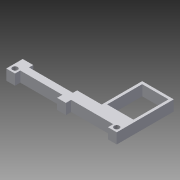
# Autodesk Inventor part: yCarMid_d
Saved by Autodesk Inventor 2013 (Build 170138000, 138)
## iProperties
Created: 2015-01-14
Part Number: yCarMid_d
Material: Generic
Document SubType Name: Modeling
Designer: dzban
Density: 1 g/cm^3
Author: dzban
Autodesk Inventor part; units mm, degrees
ref_plane "YZ Plane" through (0, 0, 0) normal (1, 0, 0) x (0, 1, 0)
ref_plane "XZ Plane" through (0, 0, 0) normal (0, 1, 0) x (-1, 0, 0)
ref_plane "XY Plane" through (0, 0, 0) normal (0, 0, 1) x (1, 0, 0)
sketch "Sketch1" plane through (0, 0, 0) normal (0, 0, 1) x (1, 0, 0)
  line L0 (46.5, 31) -> (61.5, 31)
  line L1 (61.5, 31) -> (61.5, 11)
  line L2 (61.5, 11) -> (46.5, 11)
  line L3 (46.5, 11) -> (46.5, 31)
  circle A0 centre (60.5, 2.5) radius 1.5
  circle A1 centre (2.5, 2.5) radius 1.5
  line L4 (0, 9.4) -> (0, 0)
  line L5 (0, 0) -> (5, 0)
  line L6 (5, 0) -> (5, 3)
  line L7 (5, 3) -> (29, 3)
  line L8 (29, 3) -> (29, 0)
  line L9 (29, 0) -> (34, 0)
  line L10 (34, 0) -> (34, 3)
  line L11 (34, 3) -> (58, 3)
  line L12 (58, 3) -> (58, 0)
  line L13 (58, 0) -> (63, 0)
  line L14 (63, 0) -> (63, 32.5)
  line L15 (63, 32.5) -> (45, 32.5)
  line L16 (45, 32.5) -> (45, 9.4)
  line L17 (45, 9.4) -> (31, 9.4)
  line L18 (31, 9.4) -> (31, 7)
  line L19 (31, 7) -> (6, 7)
  line L20 (6, 7) -> (6, 9.4)
  line L21 (6, 9.4) -> (0, 9.4)
  constraints: 44 end point, 2 centre point
extrude "Extrusion1" add sketch "Sketch1" along normal blind 6
body "Solid1"
